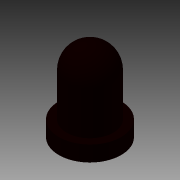
# Autodesk Inventor part: LTR_4206E_Photodiode
Saved by Autodesk Inventor 2014 (Build 180170000, 170)
## iProperties
Created: 2013-11-15
Part Number: LTR_4206E_Photodiode
Material: Generic
Document SubType Name: Modeling
Designer: Rex
Density: 1 g/cm^3
Appearance: Default
Author: Rex
Autodesk Inventor part; units mm, degrees
ref_plane "YZ Plane" through (0, 0, 0) normal (1, 0, 0) x (0, 1, 0)
ref_plane "XZ Plane" through (0, 0, 0) normal (0, 1, 0) x (-1, 0, 0)
ref_plane "XY Plane" through (0, 0, 0) normal (0, 0, 1) x (1, 0, 0)
sketch "Sketch1" plane through (0, 0, 0) normal (0, 1, 0) x (-1, 0, 0)
  circle A0 centre (-0.2574, 0.2179) radius 1.5
  point P0 (0, 0)
  dimension "d0" = 3
  constraints: 1 centre point
  measures "d0" diameter of A0
extrude "Extrusion1" add sketch "Sketch1" along normal blind 5.25
fillet "Fillet1" radius 1.5 1 edges at (1.7574, 5.25, 0.2179)
sketch "Sketch2" plane through (0, 0, 0) normal (0, 1, 0) x (-1, 0, 0)
  circle A0 centre (-0.2574, 0.2179) radius 2
  circle A1 centre (-0.2574, 0.2179) radius 1.5 projected
  circle A2 centre (-0.2574, 0.2179) radius 1.5
  point P0 (0, 0)
  dimension "d4" = 0
  dimension "d5" = 4
  dimension "d6" = 0.5
  constraints: 2 centre point, 1 coincident, 1 concentric
  measures "d4" distance of A0.centre A1.centre
  measures "d5" diameter of A0
  measures "d6" radial gap between concentric circles of A0 A1
extrude "Extrusion2" add sketch "Sketch2" along normal blind 1
body "Solid1"
